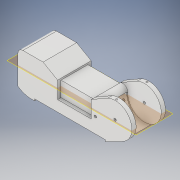
# Autodesk Inventor part: Part3
Saved by Autodesk Inventor 2017 SP1 (Build 210196100, 196)
## iProperties
Created: 2017-05-10
Part Number: Part3
Material: ABS Plastic
Document SubType Name: Modeling
Designer: zallen
Density: 1.06 g/cm^3
Appearance: Smooth - White
Mass: 1585.78 g
Surface Area: 1073.19 cm^2
Volume: 1496.02 cm^3
Author: zallen
Autodesk Inventor part; units mm, degrees
ref_plane "YZ Plane" through (0, 0, 0) normal (1, 0, 0) x (0, 1, 0)
ref_plane "XZ Plane" through (0, 0, 0) normal (0, 1, 0) x (-1, 0, 0)
ref_plane "XY Plane" through (0, 0, 0) normal (0, 0, 1) x (1, 0, 0)
sketch "Sketch1" plane through (0, 0, 0) normal (0, 0, 1) x (1, 0, 0)
  line L0 (75, 62.5) -> (0, 62.5)
  line L1 (0, 62.5) -> (0, -37.5)
  line L2 (75, 62.5) -> (118.3013, 37.5)
  line L3 (118.3013, 37.5) -> (218.3013, 37.5)
  line L4 (118.3013, 37.5) -> (218.3013, 37.5) construction
  line L5 (218.3013, 37.5) -> (268.3013, 66.3675)
  line L6 (260.727, -50) -> (50, -50)
  arc A0 (0, -37.5) -> (50, -50) centre (42.0827, 24.5809) ccw
  line L7 (260.727, -50) -> (310.727, -24.1867)
  line L8 (310.727, -24.1867) -> (268.3013, 66.3675) construction
  arc A1 (310.727, -24.1867) -> (268.3013, 66.3675) centre (289.5141, 21.0904) ccw
  point P0 (0, 0)
  point P1 (28.3617, -0.0631)
  dimension "d60" = 75
  dimension "d61" = 90
  dimension "d62" = 100
  dimension "d64" = 50
  dimension "d65" = 150
  dimension "d66" = 100
  dimension "d67" = 0
  dimension "d68" = 50
  dimension "d69" = 75
  dimension "d87" = 37.5
  dimension "d88" = 87.5
  dimension "d92" = 50
  dimension "d93" = 50
  dimension "d94" = 150
  dimension "d95" = 50
  constraints: 19 end point, 4 point on circle, 3 horizontal, 2 centre point, 1 collinear, 1 midpoint, 1 point on line, 1 vertical alignment
  measures "d60" distance of L0.end L0.start
  measures "d61" angle of L0 L1
  measures "d62" distance of L0.end L1.end
  measures "d64" distance of L0.start L2.end
  measures "d65" angle of L2 L0
  measures "d66" distance of L2.end L3.end
  measures "d67" distance between parallel lines of L3 L4
  measures "d68" horizontal distance of L1.end L6.end
  measures "d69" radius of A0
  measures "d87" distance of point (0, 0) L1.end
  measures "d88" distance between parallel lines of L3 L6
  measures "d92" horizontal distance of L6.start L7.end
  measures "d93" radius of A1
  measures "d94" angle of L3 L5
  measures "d95" horizontal distance of L3.end L5.end
extrude "Extrusion1" add sketch "Sketch1" along normal mid plane 100
ref_plane "Work Plane1" through (0, 0, 0) normal (0, 0, -1) x (-1, 0, 0)
sketch "Sketch5" plane through (0, 0, 0) normal (0, 0, -1) x (-1, 0, 0)
  circle A0 centre (-289.5141, 21.0904) radius 50
  arc A1 (-268.3013, 66.3675) -> (-310.727, -24.1867) centre (-289.5141, 21.0904) ccw projected
  point P0 (0, 0)
  point P1 (-276.1097, 50)
  dimension "d46" = 100
  constraints: 1 centre point, 1 coincident
  measures "d46" diameter of A0
extrude "Extrusion6" cut sketch "Sketch5" along normal mid plane 75
sketch "Sketch6" plane through (0, -37.5, 50) normal (-1, 0, 0) x (0, 0, 1)
  circle A0 centre (-50, 50) radius 17.5
  line L0 (0, 100) -> (-100, 100) projected
  dimension "d70" = 35
  dimension "d73" = 50
  constraints: 1 centre point, 1 coincident
  measures "d70" diameter of A0
  measures "d73" distance from line of L0 point (-50, 50)
extrude "Extrusion7" add sketch "Sketch6" along normal blind 10
sketch "Sketch7" plane through (0, 0, 50) normal (0, 0, 1) x (1, 0, 0)
  line L0 (218.3013, 37.5) -> (118.3013, 37.5) projected
  line L1 (118.3013, 37.5) -> (218.3013, 37.5)
  line L2 (218.3013, 37.5) -> (218.3013, -12.5)
  line L3 (218.3013, -12.5) -> (118.3013, -12.5)
  line L4 (118.3013, -12.5) -> (118.3013, 37.5)
  point P0 (0, 0)
  dimension "d82" = 50
  constraints: 8 end point, 2 parallel, 1 horizontal, 1 perpendicular
  measures "d82" distance between parallel lines of L3 L0
extrude "Extrusion8" cut sketch "Sketch7" against normal blind 10
sketch "Sketch8" plane through (0, 0, -50) normal (0, 0, -1) x (-1, 0, 0)
  line L0 (-75, 62.5) -> (-118.3013, 37.5) projected
  line L1 (-118.3013, 37.5) -> (-218.3013, 37.5)
  line L2 (-218.3013, 37.5) -> (-218.3013, -12.5)
  line L3 (-218.3013, -12.5) -> (-118.3013, -12.5)
  line L4 (-118.3013, -12.5) -> (-118.3013, 37.5)
  point P0 (0, 0)
  point P1 (-218.3013, 37.5)
  dimension "d84" = 50
  constraints: 8 end point, 2 parallel, 1 coincident, 1 horizontal, 1 perpendicular
  measures "d84" distance between parallel lines of L3 L1
extrude "Extrusion9" cut sketch "Sketch8" against normal blind 10
fillet "Fillet9" radius 15 1 edges at (0, 62.5, 0)
sketch "Sketch9" plane through (118.3013, 37.5, 40) normal (0, 1, 0) x (1, 0, 0)
  line L0 (0, 90) -> (0, 80) projected
  line L1 (100, 0) -> (0, 0) projected
  line L2 (0, 80) -> (100, 80)
  line L3 (100, 80) -> (100, 0)
  line L4 (100, 0) -> (0, 0)
  line L5 (0, 0) -> (0, 80)
  point P0 (-118.3013, 40)
  constraints: 8 end point, 2 parallel, 1 horizontal, 1 perpendicular
extrude "Extrusion10" cut sketch "Sketch9" against normal blind 5
fillet "Fillet10" radius 15 1 edges at (260.9094, 62.0998, 0)
sketch "Sketch10" plane through (-10, 12.5, 0) normal (-1, 0, 0) x (0, 0, 1)
  circle A0 centre (0, 0) radius 2.5
  point P0 (0, -12.5)
  dimension "d99" = 5
  constraints: 1 centre point
  measures "d99" diameter of A0
extrude "Extrusion11" cut sketch "Sketch10" against normal blind 10
sketch "Sketch11" plane through (0, 0, 0) normal (0, 0, 1) x (1, 0, 0)
  circle A0 centre (-5, 12.5) radius 2
  point P0 (0, 0)
  dimension "d102" = 4
  dimension "d103" = 12.5
  dimension "d104" = 5
  constraints: 1 centre point
  measures "d102" diameter of A0
  measures "d103" vertical distance of point (0, 0) A0.centre
  measures "d104" horizontal distance of point (0, 0) A0.centre
extrude "Extrusion12" cut sketch "Sketch11" along normal through all both and the other way through all
sketch "Sketch12" plane through (0, 0, 0) normal (0, 1, 0) x (-1, 0, 0)
  circle A0 centre (5, 0) radius 2
  point P0 (0, 0)
  dimension "d107" = 4
  dimension "d108" = 5
  constraints: 1 centre point
  measures "d107" diameter of A0
  measures "d108" distance of point (0, 0) A0.centre
extrude "Extrusion13" cut sketch "Sketch12" along normal through all both and the other way through all
sketch "Sketch13" plane through (50, -50, 50) normal (0, -1, 0) x (1, 0, 0)
  line L0 (210.727, -100) -> (0, -100) projected
  line L1 (210.727, -100) -> (210.727, 0) projected
  line L2 (0, -100) -> (210.727, -100)
  line L3 (210.727, -100) -> (210.727, 0)
  line L4 (210.727, 0) -> (0, 0)
  line L5 (0, 0) -> (0, -100)
  line L6 (10, -15) -> (205.727, -15)
  line L7 (205.727, -85) -> (10, -85)
  line L8 (10, -85) -> (10, -15)
  line L9 (205.727, -85) -> (205.727, -15)
  line L10 (218.3013, -12.5) -> (168.3013, -12.5) projected
  point P0 (-50, -50)
  dimension "d111" = 15
  dimension "d114" = 5
  dimension "d115" = 10
  dimension "d150" = 15
  constraints: 16 end point, 3 parallel, 2 perpendicular, 1 horizontal
  measures "d111" distance between parallel lines of L4 L6
  measures "d114" distance between parallel lines of L1 L9
  measures "d115" distance between parallel lines of L5 L8
  measures "d150" distance between parallel lines of L0 L7
extrude "Extrusion14" cut sketch "Sketch13" against normal blind 75 contours L6 L9 L7 L8
sketch "Sketch15" plane through (0, 0, 0) normal (0, 0, 1) x (1, 0, 0)
  line L0 (239.5315, 25) -> (60, 25) projected
  line L1 (60, -50) -> (60, 25) projected
  line L2 (110, 25) -> (60, 25)
  line L3 (60, 25) -> (60, -50)
  line L4 (60, -50) -> (110, -50)
  line L5 (110, -50) -> (110, 25)
  point P0 (0, 0)
  point P1 (118.3013, 25)
  dimension "d126" = 50
  constraints: 8 end point, 2 parallel, 1 horizontal, 1 perpendicular, 1 point on line
  measures "d126" distance between parallel lines of L1 L5
extrude "Extrusion16" add sketch "Sketch15" along normal mid plane 10
sketch "Sketch16" plane through (0, 0, -5) normal (0, 0, -1) x (-1, 0, 0)
  circle A0 centre (-97.5, -20) radius 1.65
  circle A1 centre (-97.5, 8.2843) radius 1.65
  circle A2 centre (-69.2157, -20) radius 1.65
  circle A3 centre (-69.2157, 8.2843) radius 1.65
  line L0 (-110, -50) -> (-110, 25) projected
  line L1 (-60, -50) -> (-110, -50) projected
  circle A4 centre (-83.3579, -5.8579) radius 3.5
  line L2 (-97.5, -20) -> (-69.2157, -20) construction
  line L3 (-69.2157, -20) -> (-69.2157, 8.2843) construction
  line L4 (-69.2157, 8.2843) -> (-97.5, 8.2843) construction
  line L5 (-97.5, 8.2843) -> (-97.5, -20) construction
  line L6 (-69.2157, -20) -> (-97.5, 8.2843) construction
  line L7 (-97.5, -20) -> (-69.2157, 8.2843) construction
  point P0 (0, 0)
  dimension "d129" = 3.3
  dimension "d130" = 3.3
  dimension "d131" = 3.3
  dimension "d132" = 3.3
  dimension "d133" = 28.2843
  dimension "d134" = 28.2843
  dimension "d135" = 12.5
  dimension "d136" = 30
  dimension "d139" = 7
  constraints: 12 end point, 5 centre point, 2 horizontal alignment, 2 parallel, 2 vertical alignment, 1 coincident, 1 horizontal, 1 midpoint, 1 perpendicular
  measures "d129" diameter of A0
  measures "d130" diameter of A1
  measures "d131" diameter of A2
  measures "d132" diameter of A3
  measures "d133" distance of A1.centre L2.start
  measures "d134" distance of A2.centre L2.start
  measures "d135" distance from line of L0 L2.start
  measures "d136" distance from line of L1 L2.start
  measures "d139" diameter of A4
extrude "Extrusion17" cut sketch "Sketch16" against normal blind 10
sketch "Sketch17" plane through (50, -50, 50) normal (0, -1, 0) x (1, 0, 0)
  line L0 (210.727, -100) -> (210.727, 0) projected
  line L1 (0, 0) -> (0, -100) projected
  line L2 (210.727, 0) -> (0, 0)
  line L3 (0, 0) -> (0, -100)
  line L4 (0, -100) -> (210.727, -100)
  line L5 (210.727, -100) -> (210.727, 0)
  line L6 (10, -15) -> (205.727, -15) projected
  line L7 (10, -85) -> (10, -55) projected
  line L8 (205.727, -15) -> (10, -15)
  line L9 (10, -85) -> (205.727, -85)
  line L10 (205.727, -85) -> (205.727, -15)
  line L11 (10, -15) -> (205.727, -15) projected
  line L12 (10, -45) -> (10, -15) projected
  line L13 (10, -15) -> (10, -45)
  line L14 (10, -45) -> (60, -45) projected
  line L15 (10, -45) -> (60, -45)
  line L16 (60, -45) -> (60, -55) projected
  line L17 (60, -45) -> (60, -55)
  line L18 (60, -55) -> (10, -55) projected
  line L19 (60, -55) -> (10, -55)
  line L20 (189.5315, -85) -> (10, -85) projected
  line L21 (10, -55) -> (10, -85)
  point P0 (-50, -50)
  point P1 (189.5315, -15)
  point P2 (68.3013, -90)
  dimension "d143" = 90
  constraints: 24 end point, 5 equal length, 4 perpendicular, 2 horizontal, 1 other
  measures "d143" angle of L9 L10
extrude "Extrusion18" cut sketch "Sketch17" against normal blind 5
sketch "Sketch18" plane through (50, -45, 50) normal (0, -1, 0) x (1, 0, 0)
  line L0 (10, -85) -> (205.727, -85) projected
  line L1 (10, -85) -> (60, -85)
  line L2 (60, -85) -> (60, -97)
  line L3 (60, -97) -> (10, -97)
  line L4 (10, -97) -> (10, -85)
  point P0 (-50, -50)
  dimension "d144" = 50
  dimension "d145" = 12
  constraints: 8 end point, 2 parallel, 1 horizontal, 1 perpendicular
  measures "d144" distance of L2.end L3.end
  measures "d145" distance of L1.end L2.end
extrude "Extrusion19" cut sketch "Sketch18" against normal blind 70
sketch "Sketch19" plane through (50, -45, 50) normal (0, -1, 0) x (1, 0, 0)
  line L0 (35, -45) -> (32.3579, -45)
  line L1 (29.8579, -45) -> (36.8579, -45) projected
  line L2 (36.8579, -55) -> (29.8579, -55) projected
  line L3 (29.8579, -55) -> (36.8579, -55)
  line L4 (36.8579, -55) -> (36.8579, -45)
  line L5 (36.8579, -45) -> (29.8579, -45)
  line L6 (29.8579, -45) -> (29.8579, -55)
  point P0 (-50, -50)
  constraints: 10 end point, 2 parallel, 1 horizontal, 1 perpendicular
extrude "Extrusion20" cut sketch "Sketch19" against normal blind 40
sketch "Sketch20" plane through (0, 0, 0) normal (0, 0, 1) x (1, 0, 0)
  circle A0 centre (230.8013, 0) radius 3.5
  line L0 (218.3013, -12.5) -> (218.3013, 32.5) projected
  point P0 (0, 0)
  dimension "d151" = 7
  dimension "d152" = 12.5
  constraints: 1 centre point
  measures "d151" diameter of A0
  measures "d152" distance from line of L0 A0.centre
extrude "Extrusion21" cut sketch "Sketch20" along normal through all both and the other way through all
sketch "Sketch21" plane through (50, -45, 50) normal (0, -1, 0) x (1, 0, 0)
  circle A0 centre (180.8013, -5) radius 2.5
  circle A1 centre (180.8013, -95) radius 2.5
  line L0 (184.3013, -100) -> (177.3013, -100) projected
  line L1 (177.3013, -85) -> (184.3013, -85) projected
  line L2 (29.8579, -55) -> (29.8579, -45) projected
  line L3 (10, -45) -> (29.8579, -45) projected
  line L4 (10, -15) -> (10, -45) projected
  line L5 (205.727, -15) -> (10, -15) projected
  line L6 (205.727, -85) -> (205.727, -15) projected
  line L7 (60, -85) -> (205.727, -85) projected
  line L8 (60, -85) -> (60, -97) projected
  line L9 (60, -97) -> (10, -97) projected
  line L10 (10, -97) -> (10, -55) projected
  line L11 (29.8579, -55) -> (10, -55) projected
  line L12 (0, 0) -> (210.727, 0) projected
  line L13 (0, -100) -> (0, 0) projected
  line L14 (210.727, -100) -> (0, -100) projected
  line L15 (210.727, 0) -> (210.727, -100) projected
  line L16 (184.3013, -100) -> (184.3013, -85) projected
  line L17 (177.3013, -100) -> (177.3013, -85) projected
  point P0 (-50, -50)
  dimension "d155" = 5
  dimension "d156" = 5
  dimension "d157" = 45
  dimension "d158" = 45
  constraints: 2 centre point, 1 vertical alignment
  measures "d155" diameter of A0
  measures "d156" diameter of A1
  measures "d157" vertical distance of point (-50, -50) A1.centre
  measures "d158" vertical distance of point (-50, -50) A0.centre
extrude "Extrusion22" cut sketch "Sketch21" against normal blind 50 contours A0 | A1
sketch "Sketch22" plane through (0, 0, -50) normal (0, 0, -1) x (-1, 0, 0)
  arc A0 (-268.3013, 66.3675) -> (-310.727, -24.1867) centre (-289.5141, 21.0904) ccw projected
  circle A1 centre (-289.5141, 21.0904) radius 3.5
  point P0 (0, 0)
  dimension "d161" = 7
  constraints: 1 centre point, 1 coincident
  measures "d161" diameter of A1
extrude "Extrusion23" cut sketch "Sketch22" against normal through all
ref_plane "Work Plane2" through (289.5141, 17.5904, -50) normal (0, 1, 0) x (-1, 0, 0)
sketch "Sketch25" plane through (289.5141, 17.5904, -50) normal (0, 1, 0) x (-1, 0, 0)
  circle A0 centre (0, 95) radius 2.5
  circle A1 centre (0, 5) radius 2.5
  line L0 (3.5, 87.5) -> (-3.5, 87.5) projected
  line L1 (-3.5, 100) -> (3.5, 100) projected
  line L2 (-3.5, 0) -> (-3.5, 12.5) projected
  line L3 (-3.5, 12.5) -> (3.5, 12.5) projected
  line L4 (3.5, 0) -> (3.5, 12.5) projected
  line L5 (3.5, 0) -> (-3.5, 0) projected
  line L6 (-3.5, 12.5) -> (3.5, 12.5) projected
  point P0 (289.5141, 50)
  dimension "d168" = 5
  dimension "d169" = 5
  dimension "d170" = 45
  dimension "d171" = 45
  constraints: 2 centre point
  measures "d168" diameter of A0
  measures "d169" diameter of A1
  measures "d170" vertical distance of A0.centre point (289.514, 50)
  measures "d171" vertical distance of A1.centre point (289.514, 50)
extrude "Extrusion24" cut sketch "Sketch25" along normal through all contours A0 | A1
body "Solid1"
